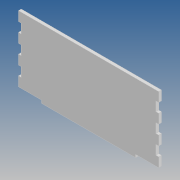
# Autodesk Inventor part: 000.104 - Back wall
Saved by Autodesk Inventor 2020 (Build 240168000, 168)
## iProperties
Created: 2021-06-28
Part Number: 000.104 - Back wall
Material: Типовые
Document SubType Name: Modeling
Designer: Петров Иван
Mass: 31.65 g
Surface Area: 225.4 cm^2
Volume: 31.65 cm^3
Density: 1 g/cm^3
Appearance: По умолчанию
Author: Петров Иван
Autodesk Inventor part; units mm, degrees
ref_plane "YZ Plane" through (0, 0, 0) normal (1, 0, 0) x (0, 1, 0)
ref_plane "XZ Plane" through (0, 0, 0) normal (0, 1, 0) x (-1, 0, 0)
ref_plane "XY Plane" through (0, 0, 0) normal (0, 0, 1) x (1, 0, 0)
sketch "Эскиз1" plane through (0, 0, 0) normal (0, 0, 1) x (1, 0, 0)
  line L0 (-74.5, -35) -> (74.5, -35)
  line L1 (74.5, -35) -> (74.5, 35)
  line L2 (74.5, 35) -> (-74.5, 35)
  line L3 (-74.5, 35) -> (-74.5, -35)
  line L4 (-74.5, -35) -> (74.5, 35) construction
  line L5 (74.5, -35) -> (-74.5, 35) construction
  point P0 (0, 0)
  dimension "d0" = 149
  dimension "d1" = 70
  constraints: 12 end point, 2 midpoint, 2 parallel, 1 horizontal, 1 perpendicular
  measures "d0" distance of L2.end L1.end
  measures "d1" distance of L1.end L0.end
extrude "Выдавливание1" add sketch "Эскиз1" along normal blind 3
sketch "Эскиз2" plane through (0, 0, 3) normal (0, 0, 1) x (1, 0, 0)
  line L0 (74.5, -35) -> (74.5, 35) projected
  line L1 (74.5, 25) -> (71.5, 25)
  line L2 (71.5, 25) -> (71.5, 15)
  line L3 (71.5, 15) -> (74.5, 15)
  line L4 (74.5, 15) -> (74.5, 25)
  line L5 (74.5, 35) -> (-74.5, 35) projected
  point P0 (0, 0)
  dimension "d4" = 3
  dimension "d5" = 10
  dimension "d6" = 10
  constraints: 8 end point, 2 parallel, 1 horizontal, 1 perpendicular, 1 point on line
  measures "d4" distance of L3.end L2.end
  measures "d5" distance of L2.end L1.end
  measures "d6" distance between parallel lines of L5 L1
extrude "Выдавливание2" cut sketch "Эскиз2" against normal blind 3
pattern_linear "Прямоуг.массив1" count 3 spacing 20 along (0, -1, 0) of "Выдавливание2"
mirror "Зеркальное отражение1" about plane through (0, 0, 0) normal (1, 0, 0) of "Выдавливание2", "Прямоуг.массив1"
sketch "Эскиз3" plane through (0, 0, 3) normal (0, 0, 1) x (1, 0, 0)
  line L0 (-74.5, -35) -> (74.5, -35) projected
  line L1 (-50, -35) -> (50, -35)
  line L2 (50, -35) -> (50, -38)
  line L3 (50, -38) -> (-50, -38)
  line L4 (-50, -38) -> (-50, -35)
  line L5 (0, 0) -> (0, -8.2609)
  line L6 (-74.5, -25) -> (-74.5, -35) projected
  dimension "d12" = 3
  dimension "d13" = 24.5
  constraints: 10 end point, 2 parallel, 1 horizontal, 1 perpendicular, 1 point on line, 1 vertical, 1 other
  measures "d12" distance of L1.end L2.end
  measures "d13" distance between parallel lines of L6 L4
extrude "Выдавливание3" add sketch "Эскиз3" against normal blind 3
